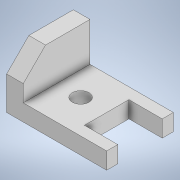
# Autodesk Inventor part: Assignment 3.6 - L-Bracket
Saved by Autodesk Inventor 2022 (Build 260153000, 153)
## iProperties
Created: 2021-05-24
Part Number: Assignment 3.6 - L-Bracket
Material: Generic
Document SubType Name: Modeling
Designer: Aaron
Density: 1 g/cm^3
Appearance: Default
Author: Aaron
Autodesk Inventor part; units mm, degrees
ref_plane "YZ Plane" through (0, 0, 0) normal (1, 0, 0) x (0, 1, 0)
ref_plane "XZ Plane" through (0, 0, 0) normal (0, 1, 0) x (-1, 0, 0)
ref_plane "XY Plane" through (0, 0, 0) normal (0, 0, 1) x (1, 0, 0)
sketch "Sketch1" plane through (0, 0, 0) normal (0, 0, 1) x (1, 0, 0)
  line L0 (0, 0) -> (114.3, 0)
  line L1 (0, 0) -> (0, 63.5)
  line L2 (0, 63.5) -> (19.05, 63.5)
  line L3 (114.3, 0) -> (114.3, 19.05)
  line L4 (114.3, 19.05) -> (19.05, 19.05)
  line L5 (19.05, 19.05) -> (19.05, 63.5)
  dimension "d0" = 114.3
  dimension "d1" = 63.5
  dimension "d2" = 19.05
  dimension "d3" = 19.05
  constraints: 12 end point, 3 perpendicular, 2 vertical, 1 horizontal
  measures "d0" distance of L0.start L0.end
  measures "d1" distance of L0.start L1.end
  measures "d2" distance of L1.end L2.end
  measures "d3" distance of L0.end L3.end
extrude "Extrusion1" add sketch "Sketch1" against normal blind 76.2
sketch "Sketch2" plane through (19.05, 19.05, 0) normal (1, 0, 0) x (0, 0, -1)
  line L0 (76.2, -19.05) -> (76.2, 44.45) projected
  line L1 (0, 44.45) -> (76.2, 44.45) projected
  line L2 (25.4, 44.45) -> (0, 44.45)
  line L3 (0, 44.45) -> (0, 19.05)
  line L4 (0, 44.45) -> (0, -19.05) projected
  line L5 (0, 19.05) -> (25.4, 44.45)
  dimension "d7" = 25.4
  constraints: 6 end point, 2 point on line
  measures "d7" distance of L1.start L3.end
extrude "Extrusion2" cut sketch "Sketch2" against normal through all
sketch "Sketch3" plane through (114.3, 0, 0) normal (1, 0, 0) x (0, 0, -1)
  line L0 (12.7, 19.05) -> (12.7, 0)
  line L1 (0, 0) -> (76.2, 0) projected
  line L2 (12.7, 19.05) -> (63.5, 19.05)
  line L3 (0, 19.05) -> (76.2, 19.05) projected
  line L4 (63.5, 19.05) -> (63.5, 0)
  line L5 (12.7, 0) -> (63.5, 0)
  dimension "d11" = 50.8
  constraints: 8 end point, 3 point on line, 2 perpendicular
  measures "d11" distance of L0.start L2.end
extrude "Extrusion3" cut sketch "Sketch3" against normal blind 38.1
sketch "Sketch4" plane through (19.05, 19.05, 0) normal (0, 1, 0) x (1, 0, 0)
  line L0 (95.25, 0) -> (0, 0) projected
  line L1 (95.25, 0) -> (95.25, 12.7) projected
  point P0 (-19.05, 0)
  point P1 (27.432, 38.1)
  dimension "d14" = 38.1
  dimension "d15" = 67.818
  measures "d14" distance from line of L0 point (27.432, 38.1)
  measures "d15" distance from line of L1 point (27.432, 38.1)
hole "Hole1" at (46.482, 19.05, -38.1) direction (0, -1, 0) diameter 19.05 end through all
body "Solid1"
